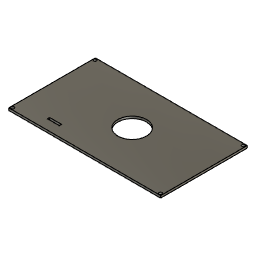
Solar Tracker Box Lid (Autodesk Fusion 360 design; units mm, degrees)
Autodesk Fusion 360 part; units mm, degrees
box "BoxPrimitive1" add length 114.7318 width 198.2216 height 2.921 placed x (0, -1, 0) y (1, 0, 0) z (0, 0, 1) at (0, 0, 0)
hole "Hole1" at (2.363, -112.1124, 2.921) direction (0, 0, -1) diameter 4 depth 50.8 tip angle 180
delete_face "DeleteFace1" 1 faces at (0.3636, -112.0625, 1.9473)
hole "Hole2" at (2.4516, -112.0641, 2.921) direction (0, 0, -1) diameter 3.9878 depth 50.8 tip angle 180
hole "Hole3" at (2.4945, -2.7892, 2.921) direction (0, 0, -1) diameter 3.9878 depth 50.8 tip angle 180
hole "Hole4" at (195.453, -111.8961, 2.921) direction (0, 0, -1) diameter 3.9878 depth 50.8 tip angle 180
hole "Hole5" at (195.4876, -2.7037, 2.921) direction (0, 0, -1) diameter 3.9878 depth 50.8 tip angle 180
hole "Hole6" at (121.7426, -60.6912, 2.921) direction (0, 0, -1) diameter 41.91 depth 50.8 tip angle 180
sketch "Sketch2" plane through (0, 0, 2.921) normal (0, 0, 1) x (-1, 0, 0)
  circle A0 centre (-121.7426, 60.6912) radius 20.955
  circle A1 centre (-195.4876, 2.7037) radius 1.9939
  circle A2 centre (-195.453, 111.8961) radius 1.9939
  circle A3 centre (-2.4945, 2.7892) radius 1.9939
  circle A4 centre (-2.4516, 112.0641) radius 1.9939
  line L0 (0, 114.7318) -> (-198.2216, 114.7318)
  line L1 (-198.2216, 114.7318) -> (-198.2216, 0)
  line L2 (-198.2216, 0) -> (0, 0)
  line L3 (0, 0) -> (0, 114.7318)
  line L4 (-38.1023, 101.602) -> (-53.9773, 101.602)
  line L5 (-53.9773, 101.602) -> (-53.9773, 98.7371)
  line L6 (-53.9773, 98.7371) -> (-38.1023, 98.7371)
  line L7 (-38.1023, 98.7371) -> (-38.1023, 101.602)
  dimension "d24" = 15.875
  constraint horizontal L4
  constraint vertical L5
  constraint horizontal L6
  constraint vertical L7
  measures "d24" distance of L4.start L4.end
extrude "Extrude1" cut sketch "Sketch2" against normal blind 34.1122 contours L4 L5 L6 L7
extrude "Extrude2" add 1 faces at (198.2216, -38.2439, 0.9737) along direction (1, 0, 0) blind 3
delete_face "DeleteFace2" 1 faces at (196.5273, -1.0023, 1.9473)
delete_face "DeleteFace3" 1 faces at (196.4927, -110.1948, 1.9473)
hole "Hole7" at (198.8061, -2.6168, 2.921) direction (0, 0, -1) diameter 4 depth 27.94 tip angle 180
hole "Hole8" at (198.6532, -112.2428, 2.921) direction (0, 0, -1) diameter 3.9878 depth 27.94 tip angle 180
hole "Hole9" at (104.6012, -55.8345, 2.921) direction (0, 0, -1) diameter 38.1 depth 27.94 tip angle 180
delete_face "DeleteFace4" 1 faces at (117.9617, -40.0801, 1.9473)
delete_face "DeleteFace5" 1 faces at (198.9058, -4.6143, 1.9473)
hole "Hole10" at (198.6413, -2.5901, 2.921) direction (0, 0, -1) diameter 4 depth 15.24 tip angle 180
